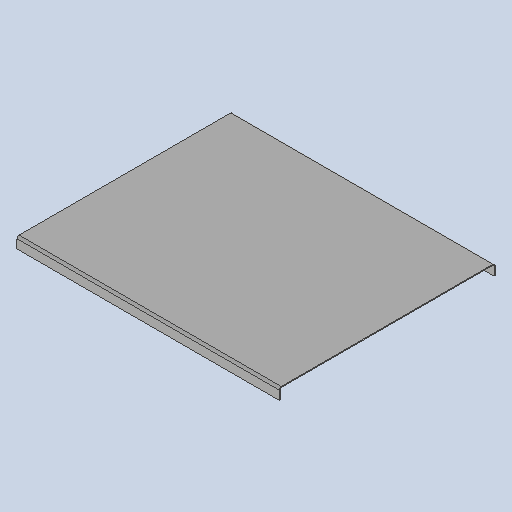
# Autodesk Inventor part: TRM 025 left board damper
Saved by Autodesk Inventor 2025 (Build 290162010, 162A)
## iProperties
Created: 2024-08-07
Part Number: TRM 025 left board damper
Material: AISI 304
Document SubType Name: Sheet Metal
Designer: pokla
Density: 8.02768 g/cm^3
Flat Pattern Width: 60 cm
Flat Pattern Length: 53.6404 cm
Flat Pattern Area: 3218.42 cm^2
Sheet Metal Rule: AISI304 2mm Die16
Sheet Metal Width: 600.000 mm
Sheet Metal Length: 536.404 mm
Sheet Metal Area: 321842.389 mm^2
Appearance: Default
Stock Number: ТРМ 025 левый борт успокоитель
Mass: 5170.93 g
Surface Area: 6486.84 cm^2
Volume: 644.137 cm^3
Author: pokla
Autodesk Inventor part; units mm, degrees
ref_plane "YZ Plane" through (0, 0, 0) normal (1, 0, 0) x (0, 1, 0)
ref_plane "XZ Plane" through (0, 0, 0) normal (0, 1, 0) x (-1, 0, 0)
ref_plane "XY Plane" through (0, 0, 0) normal (0, 0, 1) x (1, 0, 0)
sketch "Sketch1" plane through (0, 0, 0) normal (0, 0, 1) x (1, 0, 0)
  line L0 (-300, -245) -> (300, -245)
  line L1 (300, -245) -> (300, 245)
  line L2 (300, 245) -> (-300, 245)
  line L3 (-300, 245) -> (-300, -245)
  line L4 (-300, -245) -> (300, 245) construction
  line L5 (300, -245) -> (-300, 245) construction
  point P0 (0, 0)
  dimension "d0" = 600
  dimension "d1" = 490
  measures "d0" distance of L2.end L1.end
  measures "d1" distance of L1.end L0.end
extrude "Plate1" add sketch "Sketch1" along normal blind 2
sketch "Sketch2" plane through (0, 0, 0) normal (0, 0, -1) x (-1, 0, 0)
  line L0 (-280, 225) -> (-80, 225) construction
  line L1 (-80, 225) -> (-80, 205) construction
  line L2 (-80, 205) -> (-280, 205) construction
  line L3 (-280, 205) -> (-280, 225) construction
  line L4 (-300, 245) -> (300, 245) projected
  line L5 (-300, -245) -> (-300, 245) projected
  point P0 (0, 0)
  point P1 (-48, 100)
  point P2 (300, 245)
  point P3 (-50, 98)
  dimension "d6" = 200
  dimension "d9" = 20
  dimension "d10" = 20
  dimension "d11" = 20
  constraints: 4 other
  measures "d6" distance of L0.start L0.end
  measures "d9" distance of L0.end L1.end
  measures "d11" length of L3
mark "Mark1"
sketch "Sketch3" plane through (-300, 247, 2) normal (0, -1, 0) x (1, 0, 0)
  line L0 (600, 0) -> (0, 0)
  line L1 (0, 0) -> (0, 25)
  line L2 (0, 25) -> (600, 25)
  line L3 (600, 25) -> (600, 0)
  constraints: 8 end point
edge flange "Flange1" height 25 angle 90 thickness 2 bend radius 2.75 thickness toward (0, -1, 0) relief round relief width 2 relief depth 1 corner gap 2.75 corner form 0 edges at (0, 245, 2) (0, -245, 2) wall of the first edge with corners at (300, 247, 2) (-300, 247, 2) (-300, 247, -23) (300, 247, -23)
bend "Bend1"
corner "Corner1"
equation "\"d2\" = Thickness"
equation "\"d12\" = BendReliefWidth"
equation "\"d13\" = BendReliefDepth"
equation "\"d14\" = MinimumRemnant"
equation "\"d15\" = TransitionRadius"
equation "\"d18\" = BendRadius"
equation "\"d19\" = CornerReliefSize"
equation "\"d20\" = GapSize"
equation "\"d21\" = JacobiRadiusSize"
equation "\"BendReliefWidth\" = Thickness"
equation "\"BendReliefDepth\" = 0.5 * Thickness"
equation "\"CornerReliefSize\" = 4 * Thickness"
equation "\"MinimumRemnant\" = 2 * Thickness"
equation "\"TransitionRadius\" = BendRadius"
equation "\"JacobiRadiusSize\" = BendRadius"
equation "\"GapSize\" = Thickness"
equation "\"Thickness\" = 2"
equation "\"BendRadius\" = 2.75"
body "Solid1"
